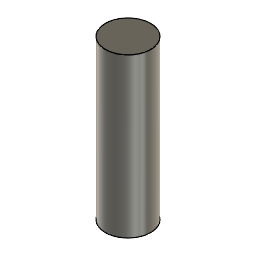
Tugboat Annie Conjugated Gear Model Assembly (Autodesk Fusion 360 archive; units mm, degrees)
design "pin 7/16"
Autodesk Fusion 360 part; units mm, degrees
sketch "Sketch1" plane through (0, 0, 0) normal (0, 0, 1) x (1, 0, 0)
  circle A0 centre (0, 0) radius 1.5875
  dimension "d1" = 3.175
  constraint coincident A0.centre origin
  measures "d1" diameter of A0
extrude "Extrude1" add sketch "Sketch1" along normal blind 11.1125
equation "d1 = ( 1 / 8 ) * 1 in"
equation "d2 = ( 7 / 16 ) * 1 in"

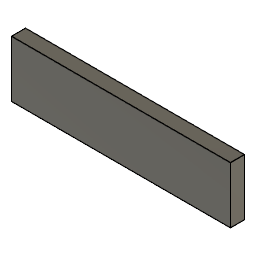
design "Frame Plate Support Bar"
Autodesk Fusion 360 part; units mm, degrees
sketch "Sketch1" plane through (0, 0, 0) normal (0, 0, 1) x (1, 0, 0)
  line L0 (0, 0) -> (49.2125, 0)
  line L1 (49.2125, 0) -> (49.2125, 3.175)
  line L2 (49.2125, 3.175) -> (0, 3.175)
  line L3 (0, 3.175) -> (0, 0)
  dimension "d1" = 49.2125
  dimension "d2" = 3.175
  constraint horizontal L0
  constraint vertical L1
  constraint horizontal L2
  constraint vertical L3
  constraint coincident L0.start L3.end
  measures "d1" distance of L0.start L0.end
  measures "d2" distance of L0.start L2.end
extrude "Extrude1" add sketch "Sketch1" along normal blind 12.7
equation "d1 = 1 15/16\""
equation "d2 = ( 1 / 8 ) * 1 in"
equation "d3 = ( 1 / 2 ) * 1 in"

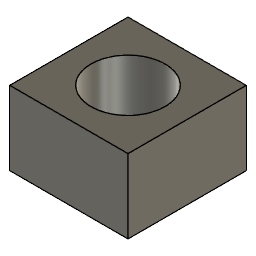
design "Die Block"
Autodesk Fusion 360 part; units mm, degrees
sketch "Sketch1" plane through (0, 0, 0) normal (0, 0, 1) x (1, 0, 0)
  line L0 (2.54, 2.54) -> (-2.54, 2.54)
  line L1 (-2.54, 2.54) -> (-2.54, -2.54)
  line L2 (-2.54, -2.54) -> (2.54, -2.54)
  line L3 (2.54, -2.54) -> (2.54, 2.54)
  line L4 (2.54, 2.54) -> (-2.54, -2.54) construction
  line L5 (-2.54, 2.54) -> (2.54, -2.54) construction
  circle A0 centre (0, 0) radius 1.5875
  dimension "d1" = 5.08
  dimension "d2" = 5.08
  dimension "d3" = 3.175
  constraint horizontal L0
  constraint perpendicular L0 L1
  constraint parallel L0 L2
  constraint parallel L1 L3
  constraint coincident L4 A0.centre
  constraint coincident L5 A0.centre
  constraint coincident A0.centre origin
  measures "d1" distance of L1.end L2.end
  measures "d2" distance of L0.end L1.end
  measures "d3" diameter of A0
extrude "Extrude1" add sketch "Sketch1" along normal blind 3.175
equation "d3 = ( 1 / 8 ) * 1 in"
equation "d4 = ( 1 / 8 ) * 1 in"

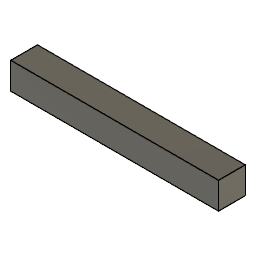
design "Frame Bracket Stand"
Autodesk Fusion 360 part; units mm, degrees
sketch "Sketch1" plane through (0, 0, 0) normal (0, 0, 1) x (1, 0, 0)
  line L0 (0, 0) -> (49.2125, 0)
  line L1 (49.2125, 0) -> (49.2125, 6.35)
  line L2 (49.2125, 6.35) -> (0, 6.35)
  line L3 (0, 6.35) -> (0, 0)
  dimension "d1" = 49.2125
  dimension "d2" = 6.35
  constraint horizontal L0
  constraint vertical L1
  constraint horizontal L2
  constraint vertical L3
  constraint coincident L0.start L3.end
  measures "d1" distance of L0.start L0.end
  measures "d2" distance of L0.start L2.end
extrude "Extrude1" add sketch "Sketch1" along normal blind 6.35
equation "d1 = 1 15/16\""
equation "d2 = ( 1 / 4 ) * 1 in"

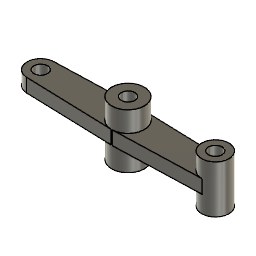
design "Equal Lever"
Autodesk Fusion 360 part; units mm, degrees
sketch "Sketch1" plane through (0, 0, 0) normal (0, 0, 1) x (1, 0, 0)
  circle A0 centre (0, 0) radius 1.5875
  line L0 (0, 0) -> (20.32, 0) construction
  line L1 (0, 0) -> (-20.32, 0) construction
  circle A1 centre (-20.32, 0) radius 1.5875
  circle A2 centre (20.32, 0) radius 1.5875
  circle A3 centre (20.32, 0) radius 3.175
  circle A4 centre (0, 0) radius 3.81
  line L2 (-0.1191, 3.8081) -> (-20.4192, 3.1734)
  line L3 (-20.4192, -3.1734) -> (-0.1191, -3.8081)
  line L4 (0.1191, -3.8081) -> (20.4192, -3.1734)
  line L5 (20.4192, 3.1734) -> (0.1191, 3.8081)
  arc A5 (-20.4192, 3.1734) -> (-20.4192, -3.1734) centre (-20.32, 0) ccw
  dimension "d1" = 3.175
  dimension "d2" = 20.32
  dimension "d3" = 20.32
  dimension "d4" = 3.175
  dimension "d5" = 3.175
  dimension "d6" = 6.35
  dimension "d7" = 6.35
  constraint coincident A0.centre L0.start
  constraint horizontal L0
  constraint parallel L0 L1
  constraint coincident L1.end A1.centre
  constraint coincident L0.end A2.centre
  constraint concentric A2 A3
  constraint concentric A1 A5
  constraint coincident A4 L2.start
  constraint coincident A4 L3.end
  constraint coincident A4 L4.start
  constraint coincident A3 L4.end
  constraint parallel L2 L4
  constraint coincident A3 L5.start
  constraint coincident A4 L5.end
  constraint tangent L2 A5
  constraint tangent L3 A5
  constraint tangent A4 L3
  constraint tangent A4 L2
  constraint tangent A4 L5
  constraint tangent A4 L4
  constraint tangent A3 L5
  measures "d1" diameter of A0
  measures "d2" distance of A0.centre L0.end
  measures "d3" distance of A0.centre L1.end
  measures "d4" diameter of A1
  measures "d5" diameter of A2
  measures "d6" diameter of A3
  measures "d7" diameter of A5
extrude "Extrude1" add sketch "Sketch1" along normal blind 1.5875 contours A3 A4 L4 L5 | A4 L2 L3 A5 makes body 1 at (-14.2982, -2.0412, 0) makes body 2 at (8.2482, 0, 0)
extrude "Extrude2" add sketch "Sketch1" along normal blind 6.35 contours A4 bodies 1 2
extrude "Extrude3" add sketch "Sketch1" along normal blind 5.5563 contours A3 bodies 1
mirror "Mirror2" about plane through (0, 0, 0) normal (0, 0, 1) of bodies 1 merged
mirror "Mirror1" [rolled back] mirror stitch tolerance 0.1016
equation "d1 = ( 1 / 8 ) * 1 in"
equation "d4 = ( 1 / 8 ) * 1 in"
equation "d5 = ( 1 / 8 ) * 1 in"
equation "d6 = ( 1 / 4 ) * 1 in"
equation "d7 = ( 1 / 4 ) * 1 in"
equation "d8 = ( 1 / 16 ) * 1 in"
equation "d10 = ( 1 / 4 ) * 1 in"
equation "d12 = ( 7 / 32 ) * 1 in"
named bodies: "Body3 (1)"

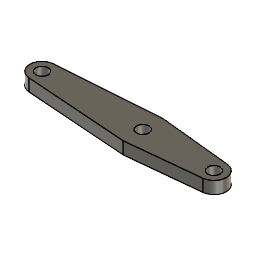
design "Ream"
Autodesk Fusion 360 part; units mm, degrees
sketch "Sketch1" plane through (0, 0, 0) normal (0, 0, 1) x (1, 0, 0)
  circle A0 centre (0, 0) radius 1.5875
  line L0 (0, 0) -> (18.415, 0) construction
  line L1 (0, 0) -> (-26.035, 0) construction
  circle A1 centre (-26.035, 0) radius 1.5875
  circle A2 centre (18.415, 0) radius 1.5875
  line L2 (0, 0) -> (0, 5.08) construction
  line L3 (0, 0) -> (0, -5.08) construction
  line L4 (0, 5.08) -> (-26.2657, 3.1666)
  line L5 (0, 5.08) -> (18.7389, 3.1584)
  line L6 (0, -5.08) -> (18.7389, -3.1584)
  line L7 (0, -5.08) -> (-26.2657, -3.1666)
  arc A3 (-26.2657, 3.1666) -> (-26.2657, -3.1666) centre (-26.035, 0) ccw
  arc A4 (18.7389, -3.1584) -> (18.7389, 3.1584) centre (18.415, 0) ccw
  dimension "d1" = 3.175
  dimension "d2" = 18.415
  dimension "d3" = 26.035
  dimension "d4" = 3.175
  dimension "d5" = 3.175
  dimension "d6" = 6.35
  dimension "d7" = 6.35
  constraint coincident A0.centre L0.start
  constraint horizontal L0
  constraint parallel L0 L1
  constraint coincident L1.end A1.centre
  constraint coincident L0.end A2.centre
  constraint concentric A1 A3
  constraint concentric A2 A4
  constraint perpendicular L0 L2
  constraint perpendicular L1 L3
  constraint tangent L4 A3
  constraint tangent L5 A4
  constraint tangent L6 A4
  constraint tangent L7 A3
  measures "d1" diameter of A0
  measures "d2" distance of A0.centre L0.end
  measures "d3" distance of A0.centre L1.end
  measures "d4" diameter of A1
  measures "d5" diameter of A2
  measures "d6" diameter of A3
  measures "d7" diameter of A4
extrude "Extrude1" add sketch "Sketch1" along normal blind 3.175
equation "d1 = ( 1 / 8 ) * 1 in"
equation "d4 = ( 1 / 8 ) * 1 in"
equation "d5 = ( 1 / 8 ) * 1 in"
equation "d6 = ( 1 / 4 ) * 1 in"
equation "d7 = ( 1 / 4 ) * 1 in"
equation "d8 = ( 1 / 8 ) * 1 in"

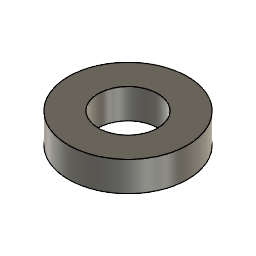
design "Washer"
Autodesk Fusion 360 part; units mm, degrees
sketch "Sketch1" plane through (0, 0, 0) normal (0, 0, 1) x (1, 0, 0)
  circle A0 centre (0, 0) radius 1.5875
  circle A1 centre (0, 0) radius 3.175
  dimension "d1" = 3.175
  dimension "d2" = 6.35
  constraint coincident A0.centre A1.centre
  measures "d1" diameter of A0
  measures "d2" diameter of A1
extrude "Extrude1" add sketch "Sketch1" along normal blind 1.5875
equation "d1 = ( 1 / 8 ) * 1 in"
equation "d2 = ( 1 / 4 ) * 1 in"
equation "d3 = ( 1 / 16 ) * 1 in"

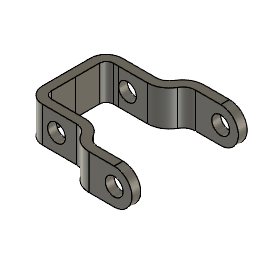
design "stirrup link"
Autodesk Fusion 360 part; units mm, degrees
sketch "Sketch1" plane through (0, 0, 0) normal (0, 0, 1) x (1, 0, 0)
  line L0 (1.745, 10.16) -> (1.745, -10.16) construction
  line L1 (15.2387, 10.16) -> (15.2387, -10.16) construction
  line L2 (-12.7, 1.0436) -> (24.13, 1.0436) construction
  line L3 (1.745, -10.16) -> (15.2387, -10.16) construction
  line L4 (8.4918, -10.16) -> (8.4918, 13.4123) construction
  line L5 (-6.35, 6.5999) -> (19.05, 6.5999) construction
  line L6 (-3.81, 9.7749) -> (21.0754, 9.7749) construction
  line L7 (15.2387, 9.7749) -> (18.4137, 9.7749)
  line L8 (1.745, 6.5999) -> (0.1575, 6.5999)
  line L9 (0.1575, 6.5999) -> (-0.766, 6.5957)
  line L10 (-2.0303, 5.326) -> (-2.0311, 1.0436)
  line L11 (15.2387, 9.7749) -> (15.2387, 6.5999) construction
  line L12 (1.745, 6.5999) -> (5.2882, 6.5999)
  line L13 (10.7551, 9.7749) -> (15.2387, 9.7749)
  arc A0 (-0.766, 6.5957) -> (-2.0303, 5.326) centre (-0.7603, 5.3257) ccw
  line L14 (0, 11.3624) -> (19.812, 11.3624) construction
  arc A1 (-0.7733, 8.1832) -> (-3.6178, 5.3263) centre (-0.7603, 5.3257) ccw
  line L15 (-3.6178, 5.3263) -> (-3.6186, 1.0436)
  line L16 (-0.7733, 8.1832) -> (5.2899, 8.1874)
  line L17 (10.7551, 11.3624) -> (18.4137, 11.3624)
  line L18 (18.4137, 9.7749) -> (18.4137, 11.3624)
  arc A2 (10.7551, 9.7749) -> (8.7111, 8.5878) centre (10.7551, 7.4216) ccw
  arc A3 (10.7551, 11.3624) -> (7.3322, 9.3745) centre (10.7551, 7.4216) ccw
  arc A4 (5.2899, 8.1874) -> (7.3322, 9.3745) centre (5.2882, 10.5406) ccw
  arc A5 (5.2882, 6.5999) -> (8.7111, 8.5878) centre (5.2882, 10.5406) ccw
  line L19 (-3.6178, -3.239) -> (-3.6186, 1.0436)
  line L20 (-2.0303, -3.2387) -> (-2.0311, 1.0436)
  arc A6 (-3.6178, -3.239) -> (-0.7733, -6.0959) centre (-0.7603, -3.2384) ccw
  arc A7 (-2.0303, -3.2387) -> (-0.766, -4.5084) centre (-0.7603, -3.2384) ccw
  line L21 (0.1575, -4.5126) -> (-0.766, -4.5084)
  line L22 (1.745, -4.5126) -> (0.1575, -4.5126)
  line L23 (-0.7733, -6.0959) -> (5.2899, -6.1001)
  line L24 (1.745, -4.5126) -> (5.2882, -4.5126)
  arc A8 (8.7111, -6.5005) -> (5.2882, -4.5126) centre (5.2882, -8.4534) ccw
  arc A9 (7.3322, -7.2872) -> (5.2899, -6.1001) centre (5.2882, -8.4534) ccw
  arc A10 (7.3322, -7.2872) -> (10.7551, -9.2751) centre (10.7551, -5.3344) ccw
  arc A11 (8.7111, -6.5005) -> (10.7551, -7.6876) centre (10.7551, -5.3344) ccw
  line L25 (10.7551, -9.2751) -> (18.4137, -9.2751)
  line L26 (10.7551, -7.6876) -> (15.2387, -7.6876)
  line L27 (15.2387, -7.6876) -> (18.4137, -7.6876)
  line L28 (18.4137, -7.6876) -> (18.4137, -9.2751)
  dimension "d1" = 13.4938
  dimension "d2" = 8.7313
  dimension "d3" = 5.5563
  dimension "d4" = 3.175
  dimension "d5" = 1.5875
  dimension "d6" = 1.27
  dimension "d7" = 1.5875
  dimension "d9" = -1.5875
  constraint vertical L0
  constraint vertical L1
  constraint perpendicular L1 L2
  constraint perpendicular L0 L3
  constraint midpoint L3 L4.start
  constraint perpendicular L3 L4
  constraint perpendicular L1 L5
  constraint perpendicular L1 L6
  constraint coincident L6 L7.start
  constraint coincident L1 L7.start
  constraint perpendicular L1 L7
  constraint coincident L5 L8.start
  constraint coincident L0 L8.start
  constraint perpendicular L0 L8
  constraint coincident L2 L10.end
  constraint coincident L1 L11.end
  constraint coincident L5 L11.end
  constraint tangent L6 A2
  constraint coincident L6 L13.start
  constraint tangent L9 A0
  constraint tangent L10 A0
  constraint perpendicular L4 L14
  constraint tangent L16 A4
  constraint coincident L14 L17.end
  constraint perpendicular L14 L18
  constraint coincident L5 L12.end
  constraint symmetric L2 L7.start L26.end
  constraint symmetric L2 L7.end L27.end
  constraint symmetric L2 L8.start L22.start
  constraint symmetric L2 L8.end L21.start
  constraint symmetric L2 L10.end L20.end
  constraint symmetric L2 L13.start A11.end
  constraint symmetric L2 L9.end A7.end
  constraint symmetric L2 L10.start L20.start
  constraint symmetric L2 A0 A7
  constraint symmetric L2 A1.start A6.end
  constraint symmetric L2 A1.end L19.start
  constraint symmetric L2 A1 A6
  constraint symmetric L2 L16.end L23.end
  constraint symmetric L2 L17.start A10.end
  constraint symmetric L2 L17.end L25.end
  constraint symmetric L2 A2 A11
  constraint symmetric L2 A3 A10
  constraint symmetric L2 A4 A9
  constraint symmetric L2 A2.end A8.start
  constraint symmetric L2 A5 A8
  constraint symmetric L2 L12.end L24.end
  constraint symmetric L2 A3.end A9.start
  measures "d1" distance of L0 L1
  measures "d2" distance of L2 L6
  measures "d3" distance of L2 L5
  measures "d4" distance of L7.start L7.end
  measures "d5" distance of L8.start L8.end
  measures "d6" radius of A0
  measures "d7" distance of L6 L14
extrude "Extrude1" add sketch "Sketch1" along normal blind 6.35
fillet "Fillet1" radius 3.175 4 edges at (18.4137, -8.4814, 6.35) (18.4137, -8.4814, 0) (18.4137, 10.5686, 0) (18.4137, 10.5686, 6.35)
sketch "Sketch2" plane through (0, -9.2751, 0) normal (0, -1, 0) x (1, 0, 0)
  arc A0 (15.2387, 0) -> (15.2387, 6.35) centre (15.2387, 3.175) ccw
  line L0 (15.2387, 6.35) -> (10.7551, 6.35)
  line L1 (10.7551, 6.35) -> (10.7551, 0)
  line L2 (10.7551, 0) -> (15.2387, 0)
  circle A1 centre (15.2387, 3.175) radius 1.5875
  line L3 (15.2387, 3.175) -> (1.745, 3.175) construction
  circle A2 centre (1.745, 3.175) radius 1.5875
  dimension "d14" = 3.175
  dimension "d15" = 13.4938
  dimension "d16" = 3.175
  constraint concentric A0 A1
  constraint coincident A0.centre A1.centre
  constraint parallel L0 L3
  constraint coincident L3.end A2.centre
  measures "d14" diameter of A1
  measures "d15" distance of A0.centre L3.end
  measures "d16" diameter of A2
extrude "Extrude2" cut sketch "Sketch2" against normal blind 26.67 contours A1 | A2
equation "d1 = ( 17 / 32 ) * 1 in"
equation "d2 = ( 11 / 32 ) * 1 in"
equation "d3 = ( 7 / 32 ) * 1 in"
equation "d4 = ( 1 / 8 ) * 1 in"
equation "d5 = ( 1 / 16 ) * 1 in"
equation "d7 = ( 1 / 16 ) * 1 in"
equation "d9 = ( -1 / 16 ) * 1 in"
equation "d10 = ( 1 / 4 ) * 1 in"
equation "d13 = ( 1 / 8 ) * 1 in"
equation "d14 = ( 1 / 8 ) * 1 in"
equation "d15 = ( 17 / 32 ) * 1 in"
equation "d16 = ( 1 / 8 ) * 1 in"

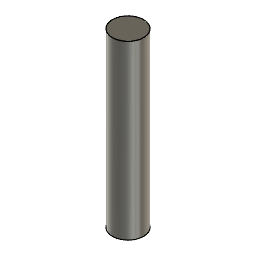
design "pin 11/16"
Autodesk Fusion 360 part; units mm, degrees
sketch "Sketch1" plane through (0, 0, 0) normal (0, 0, 1) x (1, 0, 0)
  circle A0 centre (0, 0) radius 1.5875
  dimension "d1" = 3.175
  constraint coincident A0.centre origin
  measures "d1" diameter of A0
extrude "Extrude1" add sketch "Sketch1" along normal blind 17.4625
equation "d1 = ( 1 / 8 ) * 1 in"
equation "d2 = ( 11 / 16 ) * 1 in"

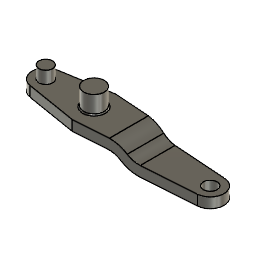
design "Cranked Lever"
Autodesk Fusion 360 part; units mm, degrees
sketch "Sketch1" plane through (0, 0, 0) normal (0, 0, 1) x (1, 0, 0)
  circle A0 centre (0, 0) radius 2.3813
  line L0 (0, 0) -> (26.924, 0) construction
  line L1 (0, 0) -> (-11.176, 0) construction
  circle A1 centre (-11.176, 0) radius 1.5875
  circle A2 centre (26.924, 0) radius 1.5875
  line L2 (0, 0) -> (0, 5.08) construction
  line L3 (0, 0) -> (0, -5.08) construction
  line L4 (0, 5.08) -> (-11.6976, 3.1319)
  line L5 (0, 5.08) -> (27.1472, 3.1671)
  line L6 (0, -5.08) -> (27.1472, -3.1671)
  line L7 (0, -5.08) -> (-11.6976, -3.1319)
  arc A3 (-11.6976, 3.1319) -> (-11.6976, -3.1319) centre (-11.176, 0) ccw
  arc A4 (27.1472, -3.1671) -> (27.1472, 3.1671) centre (26.924, 0) ccw
  dimension "d1" = 4.7625
  dimension "d2" = 26.924
  dimension "d3" = 11.176
  dimension "d4" = 3.175
  dimension "d5" = 3.175
  dimension "d6" = 6.35
  dimension "d7" = 6.35
  constraint coincident A0.centre L0.start
  constraint horizontal L0
  constraint parallel L0 L1
  constraint coincident L1.end A1.centre
  constraint coincident L0.end A2.centre
  constraint concentric A2 A4
  constraint concentric A1 A3
  constraint perpendicular L0 L2
  constraint perpendicular L0 L3
  constraint tangent L4 A3
  constraint tangent L5 A4
  constraint tangent L6 A4
  constraint tangent L7 A3
  measures "d1" diameter of A0
  measures "d2" distance of A0.centre L0.end
  measures "d3" distance of A0.centre L1.end
  measures "d4" diameter of A1
  measures "d5" diameter of A2
  measures "d6" diameter of A4
  measures "d7" diameter of A3
extrude "Extrude1" add sketch "Sketch1" along normal blind 4.7625
extrude "Extrude2" add sketch "Sketch1" along normal blind 8.89 contours A0
extrude "Extrude3" add sketch "Sketch1" along normal blind 7.62 contours A1
chamfer "Chamfer1" distance 0.254 angle 45 1 edges at (-2.2201, 0.8611, 4.7625)
sketch "Sketch2" plane through (0, 0, 0) normal (0, 1, 0) x (1, 0, 0)
  line L0 (2.3813, -5.0165) -> (-2.3813, -5.0165) construction
  line L1 (-16.51, 0) -> (-16.51, -2.3813) construction
  line L2 (-16.51, -2.3813) -> (-16.51, -4.7625) construction
  line L3 (-16.51, 0) -> (36.2684, 0) construction
  line L4 (-16.51, -4.7625) -> (-16.51, -2.3813)
  line L5 (-16.51, -2.3813) -> (7.6728, -2.3813)
  line L6 (-16.51, -4.7625) -> (7.6728, -4.7625)
  line L7 (0, 0) -> (27.1472, 0) construction
  line L8 (14.7494, -2.3813) -> (33.02, -2.3813)
  line L9 (14.732, 0) -> (33.02, 0)
  line L10 (33.02, -2.3813) -> (33.02, 0)
  arc A0 (7.6728, -2.3813) -> (10.4913, -1.4328) centre (7.6728, 2.281) ccw
  arc A1 (7.6728, -4.7625) -> (11.9309, -3.3297) centre (7.6728, 2.281) ccw
  arc A2 (14.3325, -0.0123) -> (14.3367, 0) centre (7.6728, 2.281) ccw
  arc A3 (14.7494, -2.3813) -> (11.9309, -3.3297) centre (14.7494, -7.0435) ccw
  arc A4 (14.7494, 0) -> (10.4913, -1.4328) centre (14.7494, -7.0435) ccw
  arc A5 (8.0897, -4.7502) -> (8.0855, -4.7625) centre (14.7494, -7.0435) ccw
  line L11 (27.1472, -4.7625) -> (0, -4.7625)
  line L12 (8.0855, -4.7625) -> (33.02, -4.7625)
  line L13 (33.02, -4.7625) -> (33.02, -2.3813)
  line L14 (14.3367, 0) -> (-16.51, 0)
  line L15 (-16.51, 0) -> (-16.51, -2.3813)
  dimension "d15" = 2.3813
  dimension "d16" = 2.3813
  dimension "d18" = 14.087
  constraint perpendicular L0 L1
  constraint vertical L2
  constraint perpendicular L1 L3
  constraint concentric A0 A1
  constraint tangent L5 A0
  constraint tangent L6 A1
  constraint tangent A0 A4
  constraint tangent L7 A4
  constraint concentric A3 A4
  constraint tangent A1 A3
  constraint tangent L8 A3
  constraint coincident L3 L9.start
  constraint coincident L3 L9.end
  constraint perpendicular L9 L10
  constraint coincident L3 A2.end
  constraint coincident A2.start A4
  constraint concentric A1 A2
  constraint coincident A1 A5.start
  constraint concentric A4 A5
  constraint coincident L3 A4.start
  constraint parallel L11 L12
  constraint perpendicular L5 L15
  measures "d15" distance of L1.start L1.end
  measures "d16" distance of L1.end L2.end
  measures "d18" diameter of A4
extrude "Extrude4" cut sketch "Sketch2" along normal mid plane 15.24 contours L5 A0 A2 A4 L14 L15 | L8 A1 A3 A5 L11 L12 L13
equation "d1 = ( 3 / 16 ) * 1 in"
equation "d4 = ( 1 / 8 ) * 1 in"
equation "d5 = ( 1 / 8 ) * 1 in"
equation "d6 = ( 1 / 4 ) * 1 in"
equation "d7 = ( 1 / 4 ) * 1 in"
equation "d8 = ( 3 / 16 ) * 1 in"
equation "d15 = ( 3 / 32 ) * 1 in"
equation "d16 = ( 3 / 32 ) * 1 in"

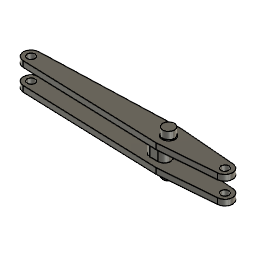
design "Big Lever"
Autodesk Fusion 360 part; units mm, degrees
sketch "Sketch1" plane through (0, 0, 0) normal (0, 0, 1) x (1, 0, 0)
  circle A0 centre (0, 0) radius 2.3812
  line L0 (0, 0) -> (22.86, 0) construction
  line L1 (0, 0) -> (-55.88, 0) construction
  circle A1 centre (-55.88, 0) radius 1.5875
  circle A2 centre (22.86, 0) radius 1.5875
  line L2 (0, 0) -> (0, 5.08) construction
  line L3 (0, 0) -> (0, -5.08) construction
  line L4 (0, 5.08) -> (-55.9881, 3.1732)
  line L5 (0, -5.08) -> (-55.9881, -3.1732)
  line L6 (0, -5.08) -> (23.1222, -3.1642)
  line L7 (0, 5.08) -> (23.1222, 3.1642)
  arc A3 (-55.9881, 3.1732) -> (-55.9881, -3.1732) centre (-55.88, 0) ccw
  arc A4 (23.1222, -3.1642) -> (23.1222, 3.1642) centre (22.86, 0) ccw
  line L8 (-55.9881, 6.509) -> (-11.5381, 6.509) construction
  line L9 (-11.5381, 6.509) -> (-11.5381, -10.8653) construction
  line L10 (-11.5381, -10.8653) -> (-55.9881, -10.8653) construction
  line L11 (-55.9881, -10.8653) -> (-55.9881, 6.509) construction
  line L12 (22.86, 0) -> (4.445, 0) construction
  line L13 (4.445, 0) -> (4.445, 12.7) construction
  line L14 (4.445, 12.7) -> (22.86, 12.7) construction
  line L15 (22.86, 12.7) -> (22.86, 0) construction
  line L16 (-5.08, 2.54) -> (-1.778, 2.54)
  line L17 (-5.08, -2.54) -> (-1.778, -2.54)
  arc A5 (-5.08, 2.54) -> (-5.08, -2.54) centre (-5.08, 0) ccw
  arc A6 (-1.778, -2.54) -> (-1.778, 2.54) centre (-1.778, 0) ccw
  dimension "d1" = 4.7625
  dimension "d2" = 22.86
  dimension "d3" = 55.88
  dimension "d4" = 3.175
  dimension "d5" = 6.35
  dimension "d6" = 3.175
  dimension "d7" = 6.35
  dimension "d8" = 44.45
  dimension "d9" = 18.415
  constraint coincident A0.centre L0.start
  constraint horizontal L0
  constraint parallel L0 L1
  constraint coincident L1.end A1.centre
  constraint concentric A1 A3
  constraint coincident L0.end A2.centre
  constraint concentric A2 A4
  constraint perpendicular L0 L2
  constraint perpendicular L1 L3
  constraint tangent L4 A3
  constraint tangent L5 A3
  constraint tangent L6 A4
  constraint tangent L7 A4
  constraint horizontal L8
  constraint vertical L9
  constraint horizontal L10
  constraint vertical L11
  constraint horizontal L12
  constraint vertical L13
  constraint horizontal L14
  constraint vertical L15
  constraint coincident L1 A5.centre
  constraint coincident L1 A6.centre
  constraint tangent L16 A6
  constraint coincident L17.start A5
  constraint tangent L17 A6
  constraint tangent L17 A5
  constraint tangent L16 A5
  constraint coincident L17 A5.end
  measures "d1" diameter of A0
  measures "d2" distance of A0.centre L0.end
  measures "d3" distance of A0.centre L1.end
  measures "d4" diameter of A1
  measures "d5" diameter of A3
  measures "d6" diameter of A2
  measures "d7" diameter of A4
  measures "d8" distance of L8.start L8.end
  measures "d9" distance of L0.end L12.end
extrude "Extrude1" add sketch "Sketch1" along normal blind 2.3813 contours A0 A6 | A0 A6 | A0 L16 L17 A5 A6 | L4 L5 L6 L7 A3 A4
extrude "Extrude2" add sketch "Sketch1" against normal blind 3.175 contours A0 A6 | A0 L16 L17 A5 A6 picked at (-0.2905, 0)
sketch "Sketch2" plane through (0, 0, 2.3813) normal (0, 0, 1) x (-1, 0, 0)
  circle A0 centre (-22.86, 0) radius 1.5875
  circle A1 centre (55.88, 0) radius 1.5875
  line L0 (0, 5.08) -> (-23.1222, 3.1642)
  arc A2 (-23.1222, 3.1642) -> (-23.1222, -3.1642) centre (-22.86, 0) ccw
  line L1 (-23.1222, -3.1642) -> (0, -5.08)
  line L2 (0, -5.08) -> (55.9881, -3.1732)
  arc A3 (55.9881, -3.1732) -> (55.9881, 3.1732) centre (55.88, 0) ccw
  line L3 (55.9881, 3.1732) -> (0, 5.08)
  circle A4 centre (0, 0) radius 2.3812
extrude "Extrude3" add sketch "Sketch2" along normal blind 3.175 contours A4
chamfer "Chamfer1" distance 0.254 angle 45 1 edges at (2.2201, -0.8611, 2.3813)
mirror "Mirror1" about plane through (0, 0, -3.175) normal (0, 0, -1) of bodies 1 merged
equation "d1 = ( 3 / 16 ) * 1 in"
equation "d4 = ( 1 / 8 ) * 1 in"
equation "d5 = ( 1 / 4 ) * 1 in"
equation "d6 = ( 1 / 8 ) * 1 in"
equation "d7 = ( 1 / 4 ) * 1 in"
equation "d10 = ( 3 / 32 ) * 1 in"
equation "d12 = ( -1 / 8 ) * 1 in"
equation "d14 = ( 4 / 32 ) * 1 in"

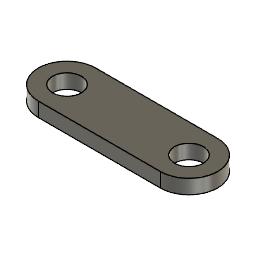
design "Link"
Autodesk Fusion 360 part; units mm, degrees
sketch "Sketch1" plane through (0, 0, 0) normal (0, 0, 1) x (1, 0, 0)
  circle A0 centre (0, 0) radius 1.5875
  line L0 (0, 0) -> (13.4938, 0) construction
  circle A1 centre (13.4938, 0) radius 1.5875
  line L1 (13.4938, 3.175) -> (0, 3.175)
  line L2 (0.0034, -3.175) -> (13.4937, -3.175)
  arc A2 (0, 3.175) -> (0.0034, -3.175) centre (0, 0) ccw
  arc A3 (13.4937, -3.175) -> (13.4938, 3.175) centre (13.4938, 0) ccw
  point P0 (13.4938, 0)
  point P1 (9.2513, -0.2613)
  dimension "d1" = 6.35
  dimension "d2" = 3.175
  dimension "d3" = 13.4938
  dimension "d4" = 6.35
  dimension "d5" = 3.175
  constraint coincident A0.centre L0.start
  constraint concentric A0 A2
  constraint horizontal L0
  constraint coincident P0 L0.end
  constraint tangent L1 A2
  constraint tangent L2 A3
  constraint tangent L1 A3
  measures "d1" diameter of A2
  measures "d2" diameter of A0
  measures "d3" distance of A0.centre P0
  measures "d4" diameter of A3
  measures "d5" diameter of A1
extrude "Extrude1" add sketch "Sketch1" along normal blind 1.5875
equation "d1 = ( 1 / 4 ) * 1 in"
equation "d2 = ( 1 / 8 ) * 1 in"
equation "d3 = ( 17 / 32 ) * 1 in"
equation "d4 = ( 1 / 4 ) * 1 in"
equation "d5 = ( 1 / 8 ) * 1 in"
equation "d6 = ( 1 / 16 ) * 1 in"

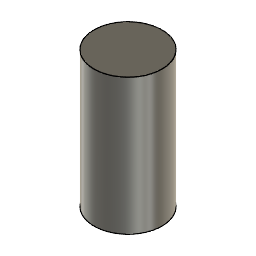
design "pin 1/4"
Autodesk Fusion 360 part; units mm, degrees
sketch "Sketch1" plane through (0, 0, 0) normal (0, 0, 1) x (1, 0, 0)
  circle A0 centre (0, 0) radius 1.5875
  dimension "d1" = 3.175
  constraint coincident A0.centre origin
  measures "d1" diameter of A0
extrude "Extrude1" add sketch "Sketch1" along normal blind 6.35
equation "d1 = ( 1 / 8 ) * 1 in"
equation "d2 = ( 1 / 4 ) * 1 in"

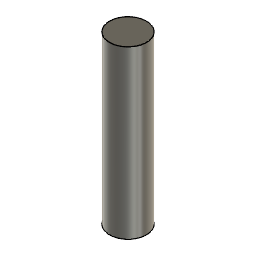
design "pin 9/16"
Autodesk Fusion 360 part; units mm, degrees
sketch "Sketch1" plane through (0, 0, 0) normal (0, 0, 1) x (1, 0, 0)
  circle A0 centre (0, 0) radius 1.5875
  dimension "d1" = 3.175
  constraint coincident A0.centre origin
  measures "d1" diameter of A0
extrude "Extrude1" add sketch "Sketch1" along normal blind 14.2875
equation "d1 = ( 1 / 8 ) * 1 in"
equation "d2 = ( 9 / 16 ) * 1 in"

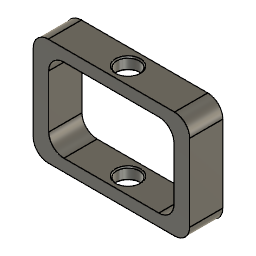
design "Cranked Lever Bracket"
Autodesk Fusion 360 part; units mm, degrees
sketch "Sketch1" plane through (0, 0, 0) normal (0, 0, 1) x (1, 0, 0)
  line L0 (0, 0) -> (32.8705, 0)
  line L1 (32.8705, 0) -> (32.8705, 6.9857)
  line L2 (32.8705, 6.9857) -> (0, 6.9857)
  line L3 (0, 6.9857) -> (0, 0)
  line L4 (0, 3.4929) -> (32.8705, 3.4929) construction
  line L5 (16.4352, 6.9857) -> (16.4352, 0) construction
  circle A0 centre (16.4352, 3.4929) radius 2.3812
  dimension "d1" = 4.7625
  constraint horizontal L0
  constraint vertical L1
  constraint horizontal L2
  constraint vertical L3
  constraint coincident L0.start L3.end
  constraint midpoint L3 L4.start
  constraint midpoint L1 L4.end
  constraint midpoint L2 L5.start
  constraint midpoint L0 L5.end
  constraint midpoint L4 A0.centre
  measures "d1" diameter of A0
extrude "Extrude1" add sketch "Sketch1" along normal blind 2.54
sketch "Sketch2" plane through (0, 0, 2.54) normal (0, 0, 1) x (-1, 0, 0)
  circle A0 centre (-16.4352, -3.4929) radius 2.3812
  line L0 (0, -6.9857) -> (0, 0)
  line L1 (0, 0) -> (-32.8705, 0)
  line L2 (-32.8705, 0) -> (-32.8705, -6.9857)
  line L3 (-32.8705, -6.9857) -> (0, -6.9857)
  line L4 (0, 0) -> (-3.2866, 0)
  line L5 (-3.2866, 0) -> (-3.2866, -6.9857)
  line L6 (-3.2866, -6.9857) -> (0, -6.9857)
  line L7 (0, -6.9857) -> (0, 0)
  line L8 (-16.4352, -3.4929) -> (-16.4352, -6.9857) construction
  line L9 (-16.4352, -3.4929) -> (-16.4352, 0) construction
  line L10 (-29.5839, 0) -> (-29.5839, -6.9857)
  line L11 (-29.5839, -6.9857) -> (-32.8705, -6.9857)
  line L12 (-32.8705, -6.9857) -> (-32.8705, 0)
  line L13 (-32.8705, 0) -> (-29.5839, 0)
  constraint horizontal L4
  constraint vertical L5
  constraint horizontal L6
  constraint vertical L7
  constraint coincident L3 L5.end
  constraint coincident L0.end L1.start
  constraint coincident A0.centre L8.start
  constraint midpoint L3 L8.end
  constraint midpoint L1 L9.end
  constraint symmetric L0.end L8 L1.end
  constraint symmetric L4.end L8 L10.start
  constraint symmetric L5.end L8 L10.end
  constraint symmetric L0.start L8 L2.end
chamfer "Chamfer1" distance 0.254 angle 45 2 edges at (14.2151, 4.354, 2.54) (14.2151, 4.354, 0)
extrude "Extrude2" add sketch "Sketch2" along normal blind 8.7313 contours L0 L1 L3 L4 L5 L6 L7 | L1 L2 L3 L10 L11 L12 L13
fillet "Fillet1" radius 3.175 4 edges at (3.2866, 3.4929, 2.54) (29.5839, 3.4929, 2.54) (32.8705, 3.4929, 0) (0, 3.4929, 0)
mirror "Mirror1" about plane through (0, 0, 11.2713) normal (0, 0, 1) of bodies 1 merged
equation "d1 = ( 3 / 16 ) * 1 in"
equation "d5 = ( 11 / 32 ) * 1 in"

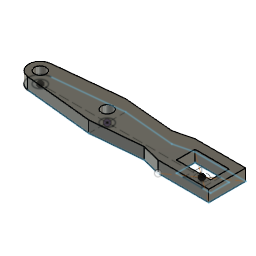
design "R.H. Rocking Lever"
Autodesk Fusion 360 part; units mm, degrees
sketch "Sketch1" plane through (0, 0, 0) normal (0, 0, 1) x (1, 0, 0)
  circle A0 centre (0, 0) radius 1.5875
  line L0 (0, 0) -> (-18.415, 0) construction
  circle A1 centre (-18.415, 0) radius 1.5875
  line L1 (0, 0) -> (0, 5.08) construction
  line L2 (0, 0) -> (0, -5.08) construction
  line L3 (0, 5.08) -> (-18.7389, 3.1584)
  line L4 (0, -5.08) -> (-18.7389, -3.1584)
  arc A2 (-18.7389, 3.1584) -> (-18.7389, -3.1584) centre (-18.415, 0) ccw
  line L5 (0, 0) -> (26.035, 0) construction
  circle A3 centre (26.035, 0) radius 1.5875 construction
  line L6 (28.575, 2.54) -> (23.495, 2.54)
  line L7 (23.495, 2.54) -> (23.495, -2.54) construction
  line L8 (23.495, -2.54) -> (28.575, -2.54)
  line L9 (28.575, -2.54) -> (28.575, 2.54) construction
  line L10 (28.575, 2.54) -> (23.495, -2.54) construction
  line L11 (23.495, 2.54) -> (28.575, -2.54) construction
  line L12 (21.59, 2.54) -> (30.988, 2.54)
  line L13 (30.988, 2.54) -> (30.988, -2.54)
  line L14 (30.988, -2.54) -> (21.59, -2.54)
  line L15 (21.59, -2.54) -> (21.59, 2.54)
  line L16 (33.02, 5.08) -> (19.05, 5.08)
  line L17 (19.05, -5.08) -> (33.02, -5.08)
  line L18 (33.02, -5.08) -> (33.02, 5.08)
  line L19 (33.02, 5.08) -> (19.05, -5.08) construction
  line L20 (19.05, 5.08) -> (33.02, -5.08) construction
  line L21 (19.05, 5.08) -> (13.97, 3.81)
  line L22 (19.05, -5.08) -> (13.97, -3.81)
  line L23 (0, 5.08) -> (13.97, 3.81)
  line L24 (0, -5.08) -> (13.97, -3.81)
  point P0 (26.035, 0)
  point P1 (26.035, 0)
  dimension "d1" = 3.175
  dimension "d2" = 18.415
  dimension "d3" = 3.175
  dimension "d4" = 6.35
  dimension "d5" = 26.035
  dimension "d6" = 3.175
  dimension "d7" = 5.08
  dimension "d12" = 5.08
  constraint coincident A0.centre L0.start
  constraint horizontal L0
  constraint coincident L0.end A1.centre
  constraint concentric A1 A2
  constraint perpendicular L0 L1
  constraint perpendicular L0 L2
  constraint tangent L3 A2
  constraint tangent L4 A2
  constraint perpendicular L2 L5
  constraint coincident P1 P0
  constraint horizontal L6
  constraint perpendicular L6 L7
  constraint parallel L6 L8
  constraint parallel L7 L9
  constraint coincident L10 P1
  constraint coincident L11 P1
  constraint horizontal L12
  constraint vertical L13
  constraint horizontal L14
  constraint vertical L15
  constraint horizontal L16
  constraint parallel L16 L17
  constraint coincident L19 P1
  constraint coincident L20 P1
  constraint symmetric L5 L16.end L17.start
  constraint symmetric L5 L21.end L22.end
  measures "d1" diameter of A0
  measures "d2" distance of A0.centre L0.end
  measures "d3" diameter of A1
  measures "d4" diameter of A2
  measures "d5" distance of A0.centre P1
  measures "d6" diameter of A3
  measures "d7" distance of L7.end L8.end
  measures "d12" distance of L6.start L8.end
extrude "Extrude1" add sketch "Sketch1" along normal blind 3.175
extrude "Extrude2" [rolled back] along distance 3.175 taper angle 0
extrude "Extrude3" [rolled back] along distance -8.89 taper angle 0
equation "d1 = ( 1 / 8 ) * 1 in"
equation "d3 = ( 1 / 8 ) * 1 in"
equation "d4 = ( 1 / 4 ) * 1 in"
equation "d6 = ( 1 / 8 ) * 1 in"
equation "d8 = ( 1 / 8 ) * 1 in"
equation "d10 = ( 1 / 8 ) * 1 in"
